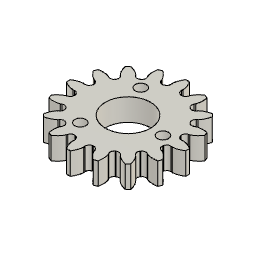
Pt_Pignon_entretoise_KOSMOS3-0 (Autodesk Fusion 360 design; units mm, degrees)
description: Spur Gear; Module: 1.5; Num Teeth: 16; Pressure Angle: 20.0; Backlash: 0.20 mm
Autodesk Fusion 360 part; units mm, degrees
note: some values were not read from the file. Set by a fixed rule: which sketch regions a step uses.
sketch "Esquisse1" plane through (0, 0, 0) normal (0, 0, 1) x (1, 0, 0) in component "Spur Gear (16 teeth)"
  circle A0 centre (0, 0) radius 10.1492
  circle A1 centre (0, 0) radius 5.1
  dimension "d15" = 10.2
  measures "d15" diameter of A1
extrude "Extrusion1" add sketch "Esquisse1" along normal blind 5 in component "Spur Gear (16 teeth)"
sketch "Esquisse2" plane through (0, 0, 0) normal (0, 0, 1) x (1, 0, 0) in component "Spur Gear (16 teeth)"
  spline S0 degree 5 poles (11.2095, -1.2257) (11.216, -1.2264) (11.229, -1.2276) (11.2485, -1.2289) (11.2747, -1.2296) (11.3074, -1.229) (11.3401, -1.2273) (11.373, -1.225) (11.4058, -1.2223) (11.4387, -1.2194) (11.4716, -1.2162) (11.5045, -1.2127) (11.5375, -1.2088) (11.5704, -1.2043) (11.6034, -1.1993) (11.6363, -1.1939) (11.6693, -1.1881) (11.7023, -1.1819) (11.7353, -1.1754) (11.7683, -1.1686) (11.8013, -1.1615) (11.8343, -1.1541) (11.8673, -1.1464) (11.9003, -1.1384) (11.9333, -1.1301) (11.9663, -1.1215) (11.9992, -1.1125) (12.0322, -1.1033) (12.0652, -1.0938) (12.0981, -1.0841) (12.131, -1.0741) (12.164, -1.0638) (12.1969, -1.0533) (12.2298, -1.0425) (12.2627, -1.0314) (12.2955, -1.0201) (12.3284, -1.0085) (12.3612, -0.9967) (12.394, -0.9846) (12.4268, -0.9723) (12.4596, -0.9598) (12.4923, -0.947) (12.525, -0.934) (12.5577, -0.9208) (12.5904, -0.9073) (12.6231, -0.8936) (12.6557, -0.8797) (12.6883, -0.8655) (12.7209, -0.8511) (12.7534, -0.8365) (12.786, -0.8217) (12.8185, -0.8067) (12.8509, -0.7914) (12.8833, -0.7759) (12.9157, -0.7603) (12.9481, -0.7444) (12.9804, -0.7283) (13.0127, -0.712) (13.045, -0.6954) (13.0772, -0.6787) (13.1094, -0.6618) (13.1416, -0.6446) (13.1737, -0.6273) (13.2058, -0.6098) (13.2378, -0.592) (13.2698, -0.5741) (13.3018, -0.5559) (13.3337, -0.5376) (13.3656, -0.5191) (13.3975, -0.5003) (13.4293, -0.4814) (13.4547, -0.4661) (13.4737, -0.4546) (13.4864, -0.4468) (13.4927, -0.4429) knots 0 0 0 0 0 0 0.01428571 0.02857143 0.04285714 0.05714286 0.07142857 0.08571429 0.1 0.11428571 0.12857143 0.14285714 0.15714286 0.17142857 0.18571429 0.2 0.21428571 0.22857143 0.24285714 0.25714286 0.27142857 0.28571429 0.3 0.31428571 0.32857143 0.34285714 0.35714286 0.37142857 0.38571429 0.4 0.41428571 0.42857143 0.44285714 0.45714286 0.47142857 0.48571429 0.5 0.51428571 0.52857143 0.54285714 0.55714286 0.57142857 0.58571429 0.6 0.61428571 0.62857143 0.64285714 0.65714286 0.67142857 0.68571429 0.7 0.71428571 0.72857143 0.74285714 0.75714286 0.77142857 0.78571429 0.8 0.81428571 0.82857143 0.84285714 0.85714286 0.87142857 0.88571429 0.9 0.91428571 0.92857143 0.94285714 0.95714286 0.97142857 0.98571429 1 1 1 1 1 1
  spline S1 degree 5 poles (11.2095, 1.2257) (11.216, 1.2264) (11.229, 1.2276) (11.2485, 1.2289) (11.2747, 1.2296) (11.3074, 1.229) (11.3401, 1.2273) (11.373, 1.225) (11.4058, 1.2223) (11.4387, 1.2194) (11.4716, 1.2162) (11.5045, 1.2127) (11.5375, 1.2088) (11.5704, 1.2043) (11.6034, 1.1993) (11.6363, 1.1939) (11.6693, 1.1881) (11.7023, 1.1819) (11.7353, 1.1754) (11.7683, 1.1686) (11.8013, 1.1615) (11.8343, 1.1541) (11.8673, 1.1464) (11.9003, 1.1384) (11.9333, 1.1301) (11.9663, 1.1215) (11.9992, 1.1125) (12.0322, 1.1033) (12.0652, 1.0938) (12.0981, 1.0841) (12.131, 1.0741) (12.164, 1.0638) (12.1969, 1.0533) (12.2298, 1.0425) (12.2627, 1.0314) (12.2955, 1.0201) (12.3284, 1.0085) (12.3612, 0.9967) (12.394, 0.9846) (12.4268, 0.9723) (12.4596, 0.9598) (12.4923, 0.947) (12.525, 0.934) (12.5577, 0.9208) (12.5904, 0.9073) (12.6231, 0.8936) (12.6557, 0.8797) (12.6883, 0.8655) (12.7209, 0.8511) (12.7534, 0.8365) (12.786, 0.8217) (12.8185, 0.8067) (12.8509, 0.7914) (12.8833, 0.7759) (12.9157, 0.7603) (12.9481, 0.7444) (12.9804, 0.7283) (13.0127, 0.712) (13.045, 0.6954) (13.0772, 0.6787) (13.1094, 0.6618) (13.1416, 0.6446) (13.1737, 0.6273) (13.2058, 0.6098) (13.2378, 0.592) (13.2698, 0.5741) (13.3018, 0.5559) (13.3337, 0.5376) (13.3656, 0.5191) (13.3975, 0.5003) (13.4293, 0.4814) (13.4547, 0.4661) (13.4737, 0.4546) (13.4864, 0.4468) (13.4927, 0.4429) knots 0 0 0 0 0 0 0.01428571 0.02857143 0.04285714 0.05714286 0.07142857 0.08571429 0.1 0.11428571 0.12857143 0.14285714 0.15714286 0.17142857 0.18571429 0.2 0.21428571 0.22857143 0.24285714 0.25714286 0.27142857 0.28571429 0.3 0.31428571 0.32857143 0.34285714 0.35714286 0.37142857 0.38571429 0.4 0.41428571 0.42857143 0.44285714 0.45714286 0.47142857 0.48571429 0.5 0.51428571 0.52857143 0.54285714 0.55714286 0.57142857 0.58571429 0.6 0.61428571 0.62857143 0.64285714 0.65714286 0.67142857 0.68571429 0.7 0.71428571 0.72857143 0.74285714 0.75714286 0.77142857 0.78571429 0.8 0.81428571 0.82857143 0.84285714 0.85714286 0.87142857 0.88571429 0.9 0.91428571 0.92857143 0.94285714 0.95714286 0.97142857 0.98571429 1 1 1 1 1 1
  arc A0 (13.4927, -0.4429) -> (13.4927, 0.4429) centre (0, 0) ccw
  line L0 (10.0791, -1.1032) -> (11.2095, -1.2257)
  line L1 (10.0791, 1.1032) -> (11.2095, 1.2257)
  line L2 (10.0791, -1.1032) -> (10.0791, 1.1032)
  point P0 (11.3693, -1.2252)
  point P1 (11.5307, -1.2095)
  point P2 (11.6931, -1.1835)
  point P3 (11.8561, -1.149)
  point P4 (12.0196, -1.1068)
  point P5 (12.1835, -1.0575)
  point P6 (12.3476, -1.0016)
  point P7 (12.5118, -0.9393)
  point P8 (12.6759, -0.8708)
  point P9 (12.84, -0.7965)
  point P10 (13.0038, -0.7164)
  point P11 (13.1672, -0.6308)
  point P12 (13.3303, -0.5396)
  point P13 (11.3693, 1.2252)
  point P14 (11.5307, 1.2095)
  point P15 (11.6931, 1.1835)
  point P16 (11.8561, 1.149)
  point P17 (12.0196, 1.1068)
  point P18 (12.1835, 1.0575)
  point P19 (12.3476, 1.0016)
  point P20 (12.5118, 0.9393)
  point P21 (12.6759, 0.8708)
  point P22 (12.84, 0.7965)
  point P23 (13.0038, 0.7164)
  point P24 (13.1672, 0.6308)
  point P25 (13.3303, 0.5396)
extrude "Extrusion2" add sketch "Esquisse2" along normal blind 5 in component "Spur Gear (16 teeth)"
fillet "Congé1" radius 0.88 2 edges at (10.0889, -1.1043, 2.5) (10.0889, 1.1043, 2.5) in component "Spur Gear (16 teeth)"
pattern_circular "Réseau C1" count 16 over 360 about axis through (0, 0, 0) along (0, 0, 1) of "Extrusion2", "Congé1" in component "Spur Gear (16 teeth)"
sketch "Esquisse3" plane through (0, 0, 0) normal (0, 0, 1) x (1, 0, 0) in component "Spur Gear (16 teeth)"
  circle A0 centre (0, 0) radius 12 construction
sketch "Esquisse1 (2)" plane through (0, 0, 0) normal (0, 0, 1) x (1, 0, 0)
  circle A0 centre (7.9, 0) radius 1.25
  circle A1 centre (-3.95, 6.8416) radius 1.25
  circle A2 centre (-3.95, -6.8416) radius 1.25
  dimension "d9" = 2.5
  dimension "d10" = 7.9
  dimension "d12" = 360
  measures "d9" diameter of A0
  measures "d10" distance of origin A0.centre
extrude "Extrusion3" cut sketch "Esquisse1 (2)" along normal blind 5 in component "Spur Gear (16 teeth)"
component "Spur Gear (16 teeth)" placed x (1, 0, 0) y (0, 1, 0) z (0, 0, 1) at (0, 0, 0)
